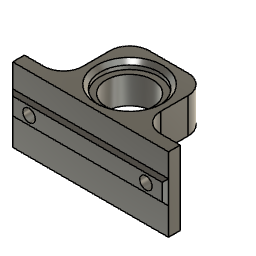
K3 power button v1 (Autodesk Fusion 360 design; units mm, degrees)
Autodesk Fusion 360 part; units mm, degrees
sketch "Sketch1" plane through (0, 0, 0) normal (0, 1, 0) x (1, 0, 0)
  line L0 (0, 0) -> (40, 0)
  line L1 (40, 0) -> (40, -20)
  line L2 (40, -20) -> (0, -20)
  line L3 (0, -20) -> (0, 0)
  dimension "d1" = 40
  dimension "d2" = 20
  constraint horizontal L0
  constraint vertical L1
  constraint horizontal L2
  constraint vertical L3
  constraint coincident L0.start L3.end
  measures "d1" distance of L0.start L0.end
  measures "d2" distance of L0.start L2.end
extrude "Extrude1" add sketch "Sketch1" along normal blind 20
sketch "Sketch2" plane through (0, 0, 20) normal (0, 0, 1) x (-1, 0, 0)
  line L0 (0, 0) -> (-40, 0)
  line L1 (-40, 0) -> (-40, -20)
  line L2 (-40, -20) -> (0, -20)
  line L3 (0, -20) -> (0, 0)
  circle A0 centre (-20, -10) radius 6
  dimension "d5" = 12
  measures "d5" diameter of A0
extrude "Extrude2" cut sketch "Sketch2" against normal blind 20 contours A0
sketch "Sketch3" plane through (0, 0, 20) normal (0, 0, 1) x (-1, 0, 0)
  circle A0 centre (-20, -10) radius 6
  line L0 (0, 0) -> (-40, 0)
  line L1 (-40, 0) -> (-40, -20)
  line L2 (-40, -20) -> (0, -20)
  line L3 (0, -20) -> (0, 0)
  circle A1 centre (-20, -10) radius 7.5
  dimension "d8" = 15
  constraint concentric A0 A1
  measures "d8" diameter of A1
extrude "Extrude3" cut sketch "Sketch3" against normal blind 2 contours A1
chamfer "Chamfer1" distance 1 angle 45 1 edges at (26.9925, 7.2879, 20)
sketch "Sketch4" plane through (0, 0, 20) normal (0, 0, 1) x (-1, 0, 0)
  line L0 (0, 0) -> (-40, 0)
  line L1 (-40, 0) -> (-40, -20)
  line L2 (-40, -20) -> (0, -20)
  line L3 (0, -20) -> (0, 0)
  circle A0 centre (-20, -10) radius 8.5
  line L4 (-40, -20) -> (-30, -20)
  line L5 (-30, -20) -> (-30, -3)
  line L6 (-30, -3) -> (-40, -3)
  line L7 (-40, -3) -> (-40, -20)
  line L8 (0, -20) -> (-10, -20)
  line L9 (-10, -20) -> (-10, -3)
  line L10 (-10, -3) -> (0, -3)
  line L11 (0, -3) -> (0, -20)
  constraint horizontal L4
  constraint vertical L5
  constraint horizontal L6
  constraint vertical L7
  constraint coincident L1.end L2.start
  constraint horizontal L8
  constraint vertical L9
  constraint horizontal L10
  constraint vertical L11
  constraint coincident L2.end L3.start
extrude "Extrude4" cut sketch "Sketch4" against normal blind 20 contours L2 L3 L8 L9 L10 L11 | L1 L2 L4 L5 L6 L7
sketch "Sketch5" plane through (0, 0, 0) normal (0, 0, -1) x (1, 0, 0)
  circle A0 centre (20, -10) radius 6
  line L0 (0, -3) -> (10, -3)
  line L1 (10, -3) -> (10, -20)
  line L2 (10, -20) -> (30, -20)
  line L3 (30, -20) -> (30, -3)
  line L4 (30, -3) -> (40, -3)
  line L5 (40, -3) -> (40, 0)
  line L6 (40, 0) -> (0, 0)
  line L7 (0, 0) -> (0, -3)
  line L8 (10, -3) -> (30, -3)
  line L9 (30, -3) -> (30, -20)
  line L10 (30, -20) -> (10, -20)
  line L11 (10, -20) -> (10, -3)
  constraint horizontal L8
  constraint vertical L9
  constraint horizontal L10
  constraint vertical L11
  constraint coincident L2.end L3.start
  constraint coincident L0.end L1.start
extrude "Extrude5" cut sketch "Sketch5" against normal blind 10 contours L1 L2 L3 L8 L9 L10 L11
sketch "Sketch6" plane through (0, 0, 10) normal (0, 0, -1) x (1, 0, 0)
  circle A0 centre (20, -10) radius 6
  line L0 (10, -20) -> (30, -20)
  line L1 (30, -20) -> (30, -3)
  line L2 (30, -3) -> (10, -3)
  line L3 (10, -3) -> (10, -20)
  circle A1 centre (20, -10) radius 9
  dimension "d16" = 18
  constraint concentric A0 A1
  measures "d16" diameter of A1
extrude "Extrude6" cut sketch "Sketch6" along normal blind 10 contours L2 A1 picked at (21.5234, -2.3453)
fillet "Fillet1" radius 5 2 edges at (27.8284, 3, 10) (12.1716, 3, 10)
sketch "Sketch7" plane through (0, 0, 0) normal (0, -1, 0) x (1, 0, 0)
  line L0 (40, 20) -> (0, 20)
  line L1 (0, 20) -> (0, 0)
  line L2 (0, 0) -> (40, 0)
  line L3 (40, 0) -> (40, 20)
  line L4 (0, 7) -> (40, 7)
  line L5 (40, 7) -> (40, 13)
  line L6 (40, 13) -> (0, 13)
  line L7 (0, 13) -> (0, 7)
  dimension "d21" = 40
  dimension "d22" = 6
  constraint horizontal L4
  constraint vertical L5
  constraint horizontal L6
  constraint vertical L7
  constraint coincident L1 L4.start
  measures "d21" distance of L4.start L4.end
  measures "d22" distance of L4.start L6.end
extrude "Extrude7" add sketch "Sketch7" along normal blind 0.8 contours L1 L3 L4 L5 L6 L7
chamfer "Chamfer2" distance 0.8 angle 45 2 edges at (20, -0.8, 7) (20, -0.8, 13)
sketch "Sketch8" plane through (0, -0.8, 0) normal (0, -1, 0) x (1, 0, 0)
  line L0 (40, 12.2) -> (0, 12.2)
  line L1 (0, 12.2) -> (0, 7.8)
  line L2 (0, 7.8) -> (40, 7.8)
  line L3 (40, 7.8) -> (40, 12.2)
  line L4 (0, 10) -> (5, 10) construction
  line L5 (40, 10) -> (35, 10) construction
  circle A0 centre (35, 10) radius 1.6
  circle A1 centre (5, 10) radius 1.6
  dimension "d26" = 5
  dimension "d27" = 5
  dimension "d28" = 3.2
  dimension "d29" = 3.2
  constraint midpoint L1 L4.start
  constraint perpendicular L1 L4
  constraint midpoint L3 L5.start
  constraint perpendicular L3 L5
  constraint coincident L5.end A0.centre
  constraint coincident L4.end A1.centre
  measures "d26" distance of L4.start L4.end
  measures "d27" distance of L5.start L5.end
  measures "d28" diameter of A0
  measures "d29" diameter of A1
extrude "Extrude8" cut sketch "Sketch8" against normal blind 3.8 contours A0 | A1
fillet "Fillet2" radius 5 2 edges at (30, 3, 12.5) (10, 3, 12.5)
sketch "Sketch9" plane through (0, 3, 0) normal (0, 1, 0) x (-1, 0, 0)
  line L0 (-35, 11.6) -> (-35, 20)
  line L1 (-35, 20) -> (-40, 20)
  line L2 (-40, 20) -> (-40, 0)
  line L3 (-40, 0) -> (-25.6569, 0)
  line L4 (-25.6569, 0) -> (-25.6569, 5)
  line L5 (-25.6569, 5) -> (-35, 5)
  line L6 (-35, 5) -> (-35, 8.4)
  arc A0 (-35, 11.6) -> (-35, 8.4) centre (-35, 10) ccw
  circle A1 centre (-35, 10) radius 3
  dimension "d34" = 6
  constraint concentric A0 A1
  measures "d34" diameter of A1
extrude "Extrude9" cut sketch "Sketch9" along normal blind 1 contours L0 L6 A0 A1 picked at (-34, 10)
sketch "Sketch10" plane through (0, 3, 0) normal (0, 1, 0) x (-1, 0, 0)
  line L0 (-5, 20) -> (-5, 11.6)
  arc A0 (-5, 8.4) -> (-5, 11.6) centre (-5, 10) ccw
  line L1 (-5, 8.4) -> (-5, 5)
  line L2 (-5, 5) -> (-14.3431, 5)
  line L3 (-14.3431, 5) -> (-14.3431, 0)
  line L4 (-14.3431, 0) -> (0, 0)
  line L5 (0, 0) -> (0, 20)
  line L6 (0, 20) -> (-5, 20)
  circle A1 centre (-5, 10) radius 3
  dimension "d37" = 6
  constraint concentric A0 A1
  measures "d37" diameter of A1
extrude "Extrude10" cut sketch "Sketch10" along normal blind 1 contours L0 A0 L1 A1 picked at (-5.9972, 9.9253)
fillet "Fillet3" radius 5 2 edges at (10, 20, 15) (30, 20, 15)
delete_face "DeleteFace1" 1 faces at (11.8435, 10.4071, 19.6667)
extrude "Extrude11" cut 1 faces at (13.0503, 10.6707, 18) along direction (0, 0, -1) blind 1
extrude "Extrude12" cut 1 faces at (20.1868, 0.8403, 20) along direction (0, 0, -1) blind 1
chamfer "Chamfer3" distance 1 angle 45 1 edges at (26.9925, 12.7121, 19)
chamfer "Chamfer4" distance 0.8 angle 45 2 edges at (0, -0.8, 10) (40, -0.8, 10)
